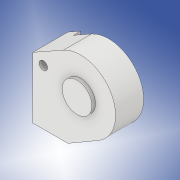
# Autodesk Inventor part: BA004
Saved by Autodesk Inventor 2017 SP1 (Build 210196100, 196)
## iProperties
Created: 2017-06-15
Part Number: BA004
Material: ABS Plastic
Document SubType Name: Modeling
Designer: zallen
Density: 1.06 g/cm^3
Appearance: CR White
Author: zallen
Autodesk Inventor part; units mm, degrees
ref_plane "YZ Plane" through (0, 0, 0) normal (1, 0, 0) x (0, 1, 0)
ref_plane "XZ Plane" through (0, 0, 0) normal (0, 1, 0) x (-1, 0, 0)
ref_plane "XY Plane" through (0, 0, 0) normal (0, 0, 1) x (1, 0, 0)
sketch "Sketch1" plane through (0, 0, 0) normal (0, 0, 1) x (1, 0, 0)
  line L0 (0, 0) -> (0, 87.5)
  circle A0 centre (68.0717, 68.3624) radius 50 construction
  line L1 (0, 87.5) -> (43.6046, 111.967)
  line L2 (0, 0) -> (50, 0)
  line L3 (50, 0) -> (93.217, 25.1454)
  arc A1 (93.217, 25.1454) -> (43.6046, 111.967) centre (68.0717, 68.3624) ccw
  dimension "d0" = 87.5
  dimension "d1" = 100
  dimension "d2" = 50
  dimension "d3" = 50
  dimension "d4" = 50
  constraints: 8 end point, 4 point on circle, 4 tangent, 2 centre point, 1 horizontal, 1 vertical
  measures "d0" distance of L0.start L0.end
  measures "d1" diameter of A0
  measures "d2" distance of L0.start L2.end
  measures "d3" distance of L0.end L1.end
  measures "d4" distance of L2.end L3.end
extrude "Extrusion1" add sketch "Sketch1" along normal blind 50
sketch "Sketch3" plane through (0, 0, 0) normal (0, 0, -1) x (-1, 0, 0)
  line L0 (0, 87.5) -> (-43.6046, 111.967) projected
  arc A0 (-43.6046, 111.967) -> (-93.217, 25.1454) centre (-68.0717, 68.3624) ccw projected
  line L1 (-93.217, 25.1454) -> (-50, 0) projected
  line L2 (-50, 0) -> (0, 0) projected
  line L3 (0, 5) -> (-48.6512, 5)
  line L4 (-48.6512, 5) -> (-90.7025, 29.4671)
  arc A1 (-46.0513, 107.6066) -> (-90.7025, 29.4671) centre (-68.0717, 68.3624) ccw
  line L5 (-46.0513, 107.6066) -> (0, 81.7667)
  line L6 (0, 0) -> (0, 87.5) projected
  line L7 (0, 5) -> (0, 81.7667)
  line L8 (0, 87.5) -> (0, 0) projected
  dimension "d10" = 5
  constraints: 8 end point, 2 point on circle, 1 centre point, 1 collinear, 1 point on line, 3 other
  measures "d10" radial gap between concentric circles of A0 A1
extrude "Extrusion3" cut sketch "Sketch3" against normal blind 45 contours L6 L3 L4 A1 L5
sketch "Sketch4" plane through (0, 0, 45) normal (0, 0, -1) x (-1, 0, 0)
  arc A0 (-43.6046, 111.967) -> (-93.217, 25.1454) centre (-68.0717, 68.3624) ccw projected
  circle A1 centre (-68.0717, 68.3624) radius 6.25
  point P0 (0, 0)
  dimension "d13" = 12.5
  constraints: 1 centre point, 1 coincident
  measures "d13" diameter of A1
extrude "Extrusion4" cut sketch "Sketch4" against normal through all
sketch "Sketch5" plane through (0, 0, 45) normal (0, 0, -1) x (-1, 0, 0)
  circle A0 centre (-68.0717, 68.3624) radius 6.25 projected
  circle A1 centre (-68.0717, 68.3624) radius 6.25
  circle A2 centre (-68.0717, 68.3624) radius 21.25
  point P0 (0, 0)
  dimension "d16" = 15
  constraints: 2 centre point, 1 coincident
  measures "d16" radial gap between concentric circles of A0 A2
extrude "Extrusion5" add sketch "Sketch5" along normal blind 35
sketch "Sketch6" plane through (0, 0, 50) normal (0, 0, 1) x (1, 0, 0)
  circle A0 centre (68.0717, 68.3624) radius 21.25 projected
  point P0 (0, 0)
extrude "Extrusion6" add sketch "Sketch6" along normal blind 5
sketch "Sketch7" plane through (0, 0, 0) normal (0, 0, -1) x (-1, 0, 0)
  arc A0 (-43.6046, 111.967) -> (-93.217, 25.1454) centre (-68.0717, 68.3624) ccw projected
  line L0 (-18.0717, 68.3624) -> (-18.0717, 97.6402)
  line L1 (0, 87.5) -> (-43.6046, 111.967) projected
  line L2 (-18.0717, 97.6402) -> (-43.6046, 111.967)
  line L3 (-68.0717, 18.3624) -> (-81.5592, 18.3624)
  line L4 (-93.217, 25.1454) -> (-50, 0) projected
  line L5 (-50, 0) -> (-93.217, 25.1454) projected
  line L6 (-81.5592, 18.3624) -> (-93.217, 25.1454)
  arc A1 (-93.217, 25.1454) -> (-68.0717, 18.3624) centre (-68.0717, 68.3624) ccw
  arc A2 (-43.6046, 111.967) -> (-93.217, 25.1454) centre (-68.0717, 68.3624) ccw projected
  arc A3 (-18.0717, 68.3624) -> (-43.6046, 111.967) centre (-68.0717, 68.3624) ccw
  circle A4 centre (-68.0717, 68.3624) radius 50
  point P0 (0, 0)
  constraints: 8 end point, 4 point on circle, 3 centre point, 2 collinear, 2 point on line, 1 coincident, 1 horizontal, 1 horizontal alignment, 1 vertical, 1 vertical alignment
extrude "Extrusion7" cut sketch "Sketch7" against normal blind 10
sketch "Sketch8" plane through (0, 0, 45) normal (0, 0, -1) x (-1, 0, 0)
  circle A0 centre (-21.5, 30) radius 5
  circle A1 centre (-21.5, 30) radius 15
  line L0 (-50, 0) -> (0, 0) projected
  line L1 (0, 0) -> (0, 5) projected
  dimension "d23" = 10
  dimension "d24" = 30
  dimension "d25" = 30
  dimension "d26" = 21.5
  constraints: 2 centre point, 1 coincident
  measures "d23" diameter of A0
  measures "d24" diameter of A1
  measures "d25" distance from line of L0 A0.centre
  measures "d26" distance from line of L1 A0.centre
extrude "Extrusion8" add sketch "Sketch8" along normal blind 45
sketch "Sketch9" plane through (0, 0, 50) normal (-1, 0, 0) x (0, 0, 1)
  line L0 (0, 87.5) -> (-50, 87.5)
  line L1 (-50, 87.5) -> (-50, 72.5)
  line L2 (-50, 72.5) -> (0, 72.5)
  line L3 (0, 72.5) -> (0, 87.5)
  line L4 (0, 87.5) -> (-15, 87.5)
  line L5 (-15, 87.5) -> (-15, 32.5)
  line L6 (-15, 32.5) -> (0, 32.5)
  line L7 (0, 32.5) -> (0, 87.5)
  line L8 (-50, 0) -> (0, 0) projected
  dimension "d29" = 50
  dimension "d30" = 15
  dimension "d31" = 15
  dimension "d32" = 32.5
  constraints: 16 end point, 4 parallel, 2 horizontal, 2 perpendicular, 1 coincident
  measures "d29" distance of L2.end L1.end
  measures "d30" distance of L1.end L0.end
  measures "d31" distance of L6.end L5.end
  measures "d32" distance between parallel lines of L8 L6
extrude "Extrusion9" add sketch "Sketch9" against normal blind 5
sketch "Sketch10" plane through (0, 0, 45) normal (0, 0, -1) x (-1, 0, 0)
  circle A0 centre (-15, 78.7167) radius 10
  circle A1 centre (-15, 78.7167) radius 6
  line L0 (-18.0717, 91.9069) -> (-5, 84.5722) projected
  line L1 (-5, 72.5) -> (-5, 84.5722) projected
  point P0 (0, 0)
  dimension "d35" = 20
  dimension "d36" = 12
  constraints: 2 centre point, 2 tangent, 1 coincident
  measures "d35" diameter of A0
  measures "d36" diameter of A1
extrude "Extrusion10" add sketch "Sketch10" along normal blind 45 contours A0
sketch "Sketch11" plane through (0, 0, 0) normal (0, 0, -1) x (-1, 0, 0)
  circle A0 centre (-15, 78.7167) radius 6 projected
  circle A1 centre (-15, 78.7167) radius 2.5
  point P0 (0, 0)
  dimension "d39" = 5
  constraints: 1 centre point, 1 coincident
  measures "d39" diameter of A1
extrude "Extrusion11" add sketch "Sketch11" against normal blind 10
sketch "Sketch13" plane through (0, 0, 50) normal (0, 0, 1) x (1, 0, 0)
  circle A0 centre (15, 78.7167) radius 6 projected
  point P0 (0, 0)
extrude "Extrusion12" cut sketch "Sketch13" against normal blind 5
body "Solid1"
